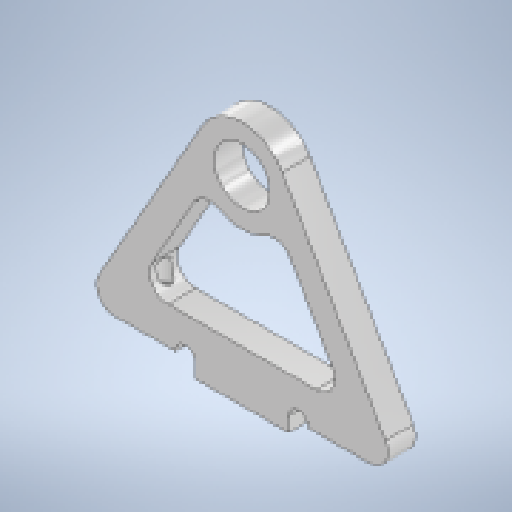
# Autodesk Inventor part: kosipiti
Saved by Autodesk Inventor 2025.1 (Build 291241000, 241)
## iProperties
Created: 2024-09-01
Part Number: kosipiti
Material: アルミニウム 2014-T4
Document SubType Name: Modeling
Designer: right
Density: 2.8 g/cm^3
Appearance: サテン
Mass: 2.41598 g
Surface Area: 11.4548 cm^2
Volume: 0.86285 cm^3
Author: right
Autodesk Inventor part; units mm, degrees
ref_plane "YZ Plane" through (0, 0, 0) normal (1, 0, 0) x (0, 1, 0)
ref_plane "XZ Plane" through (0, 0, 0) normal (0, 1, 0) x (-1, 0, 0)
ref_plane "XY Plane" through (0, 0, 0) normal (0, 0, 1) x (1, 0, 0)
sketch "スケッチ1" plane through (0, 0, 0) normal (0, 0, 1) x (1, 0, 0)
  circle A0 centre (0, 0) radius 3
  circle A1 centre (0, 0) radius 5
  line L0 (-5, -20) -> (5, -20)
  line L1 (5, -20) -> (5, -21.5)
  line L2 (5, -21.5) -> (-5, -21.5)
  line L3 (-5, -21.5) -> (-5, -20)
  circle A2 centre (-6.1, -20) radius 1.1
  line L4 (0, 0) -> (0, -20) construction
  circle A3 centre (6.1, -20) radius 1.1
  line L5 (-7.2, -20) -> (-17.2, -20)
  line L6 (-17.2, -20) -> (-4.3402, 2.4825)
  line L7 (7.2, -20) -> (17.2, -20)
  line L8 (17.2, -20) -> (4.3402, 2.4825)
  point P0 (0, -21.5)
  point P1 (4.3402, 2.4825)
  dimension "d1" = 10
  dimension "d0" = 6
  dimension "d2" = 10
  dimension "d3" = 1.5
  dimension "d4" = 2.2
  dimension "d5" = 20
  dimension "d6" = 10
  constraints: 18 end point, 4 symmetric about line, 3 centre point, 2 coincident, 2 horizontal, 2 horizontal alignment, 2 midpoint, 2 parallel, 2 point on circle, 1 perpendicular, 1 vertical alignment, 5 other
  measures "d0" diameter of A0
  measures "d2" distance of L1.end L2.end
  measures "d3" distance of L0.end L1.end
  measures "d4" diameter of A2
  measures "d5" distance from line of L0 L4.start
  measures "d6" distance of L5.start L5.end
extrude "押し出し1" add sketch "スケッチ1" along normal blind 3 contours A1 | A1 L8 L7 A3 L0 A2 L5 L6 | L1 L2 L3 L0
fillet "フィレット1" radius 2 2 edges at (-17.2, -20, 1.5) (17.2, -20, 1.5)
sketch "スケッチ3" plane through (0, 0, 0) normal (0, 0, -1) x (-1, 0, 0)
  arc A0 (-15.488, -17.007) -> (-13.752, -20) centre (-13.752, -18) ccw projected
  line L0 (-7.2, -20) -> (-13.752, -20) projected
  arc A1 (-5, -20) -> (-7.2, -20) centre (-6.1, -20) ccw projected
  line L1 (-5, -21.5) -> (-5, -20) projected
  line L2 (5, -21.5) -> (-5, -21.5) projected
  line L3 (5, -20) -> (5, -21.5) projected
  arc A2 (7.2, -20) -> (5, -20) centre (6.1, -20) ccw projected
  line L4 (13.752, -20) -> (7.2, -20) projected
  arc A3 (13.752, -20) -> (15.488, -17.007) centre (13.752, -18) ccw projected
  line L5 (4.3402, 2.4825) -> (15.488, -17.007) projected
  arc A4 (4.3402, 2.4825) -> (-4.3402, 2.4825) centre (0, 0) ccw projected
  line L6 (-15.488, -17.007) -> (-4.3402, 2.4825) projected
  circle A5 centre (0, 0) radius 3 projected
  line L7 (-11.4559, -16) -> (11.4559, -16)
  line L8 (11.4559, -16) -> (4.0113, -2.9848)
  line L9 (-11.4559, -16) -> (-4.0113, -2.9848)
  line L10 (-15.488, -17.007) -> (-4.3402, 2.4825) projected
  circle A6 centre (0, 0) radius 5
  line L11 (5, -21.5) -> (-5, -21.5) projected
  arc A7 (4.3402, 2.4825) -> (-4.3402, 2.4825) centre (0, 0) ccw projected
  point P0 (0, -21.5)
  point P1 (0, -16)
  point P2 (0, -21.5)
  dimension "d19" = 4
  dimension "d20" = 3
  constraints: 6 end point, 3 midpoint, 3 parallel, 2 point on circle, 2 vertical alignment, 1 centre point, 1 coincident, 1 concentric, 1 horizontal
  measures "d19" distance from line of A2.centre L7
  measures "d20" distance between parallel lines of L6 L9
extrude "押し出し2" cut sketch "スケッチ3" against normal through all contours A6 L8 L7 L9
fillet "フィレット2" radius 2 4 edges at (-4.0113, -2.9848, 1.5) (4.0113, -2.9848, 1.5) (-11.4559, -16, 1.5) (11.4559, -16, 1.5)
sketch "スケッチ2" plane through (-17.2, -20, 0) normal (0, -1, 0) x (1, 0, 0)
  line L0 (12.2, 0) -> (12.2, 3) projected
  line L1 (22.2, 0) -> (22.2, 3) projected
  point P0 (17.2, 0)
  point P1 (7.2, 1.5)
  point P2 (27.2, 1.5)
  point P3 (12.2, 1.5)
  point P4 (22.2, 1.5)
  point P5 (12.2, 1.5)
  point P6 (22.2, 1.5)
  dimension "d9" = 5
  dimension "d10" = 5
  constraints: 4 midpoint, 2 horizontal alignment
  measures "d9" distance of point (7.2, 1.5) point (12.2, 1.5)
  measures "d10" distance of point (27.2, 1.5) point (22.2, 1.5)
hole "穴1" at (-10, -20, 1.5) at (10, -20, 1.5) direction (0, 1, 0) diameter 1.567 depth 6.3 tip angle 118 thread size "M2x0.4" class "6H" standard "ISO Metric profile"
equation "\"d10\" = d9"
